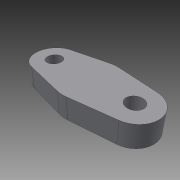
# Autodesk Inventor part: y_axis_cap
Saved by Autodesk Inventor 2014 (Build 180170000, 170)
## iProperties
Created: 2013-12-09
Part Number: y_axis_cap
Material: Generic
Document SubType Name: Modeling
Designer: buben
Density: 1 g/cm^3
Appearance: Default
Author: buben
Subject: Laser Cutted
Autodesk Inventor part; units mm, degrees
ref_plane "YZ Plane" through (0, 0, 0) normal (1, 0, 0) x (0, 1, 0)
ref_plane "XZ Plane" through (0, 0, 0) normal (0, 1, 0) x (-1, 0, 0)
ref_plane "XY Plane" through (0, 0, 0) normal (0, 0, 1) x (1, 0, 0)
sketch "Sketch1" plane through (0, 0, 0) normal (0, 0, 1) x (1, 0, 0)
  circle A0 centre (0, 0) radius 4 construction
  circle A1 centre (-12, 0) radius 2.25
  circle A2 centre (12, 0) radius 2.25
  line L0 (-12, 0) -> (0, 0) construction
  line L1 (12, 0) -> (0, 0) construction
  arc A3 (-13, 5.9161) -> (-13, -5.9161) centre (-12, 0) ccw
  arc A4 (13, -5.9161) -> (13, 5.9161) centre (12, 0) ccw
  line L2 (-13, 5.9161) -> (-1.3333, 7.8881)
  line L3 (1.3333, 7.8881) -> (13, 5.9161)
  line L4 (1.3333, -7.8881) -> (13, -5.9161)
  line L5 (-1.3333, -7.8881) -> (-13, -5.9161)
  arc A5 (1.3333, 7.8881) -> (-1.3333, 7.8881) centre (0, 0) ccw
  arc A6 (-1.3333, -7.8881) -> (1.3333, -7.8881) centre (0, 0) ccw
  circle A7 centre (-12, 0) radius 4.5 construction
  dimension "d0" = 8
  dimension "d2" = 4.5
  dimension "d3" = 8
  dimension "d4" = 12
  dimension "d5" = 9
  dimension "d6" = 6
  constraints: 12 end point, 8 centre point, 8 point on circle, 8 tangent, 5 coincident, 3 equal radius, 2 collinear, 1 horizontal
  measures "d0" diameter of A0
  measures "d2" diameter of A1
  measures "d3" radius of A6
  measures "d4" distance of L0.start L0.end
  measures "d5" diameter of A7
  measures "d6" radius of A3
extrude "Extrusion1" add sketch "Sketch1" along normal blind 6
body "Solid1"
